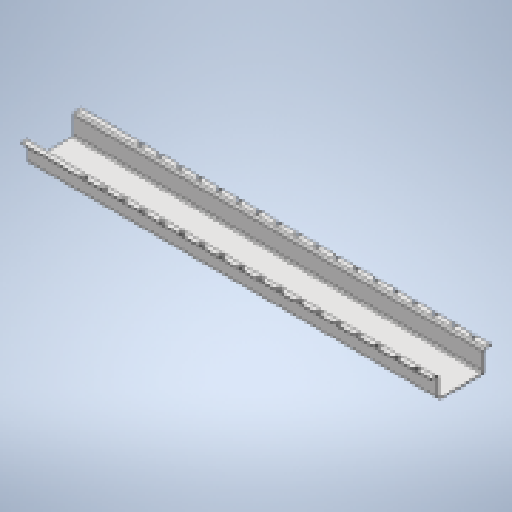
# Autodesk Inventor part: MSC 081 pillar 1_CPY
Saved by Autodesk Inventor 2025 (Build 290162010, 162A)
## iProperties
Created: 2024-06-25
Part Number: MSC 081 pillar 1_CPY
Material: Stainless Steel
Document SubType Name: Sheet Metal
Designer: admin
Density: 8 g/cm^3
Sheet Metal Rule: AISI304 3mm Die 32
Appearance: Default
Author: admin
Autodesk Inventor part; units mm, degrees
ref_plane "YZ Plane" through (0, 0, 0) normal (1, 0, 0) x (0, 1, 0)
ref_plane "XZ Plane" through (0, 0, 0) normal (0, 1, 0) x (-1, 0, 0)
ref_plane "XY Plane" through (0, 0, 0) normal (0, 0, 1) x (1, 0, 0)
sketch3d "3D Sketch1"
sketch "Sketch1" plane through (0, 0, 0) normal (0, 0, 1) x (1, 0, 0)
  line L0 (-675, 75) -> (675, 75)
  line L1 (675, 75) -> (675, -75)
  line L2 (675, -75) -> (-675, -75)
  line L3 (-675, -75) -> (-675, 75)
  line L4 (-675, 75) -> (675, -75) construction
  line L5 (675, 75) -> (-675, -75) construction
  point P0 (0, 0)
  dimension "d5" = 1350
  dimension "d30" = 150
  measures "d5" distance of L1.end L2.end
  measures "d30" distance of L2.end L0.start
extrude "Plate1" add sketch "Sketch1" along normal blind 3
sketch "Sketch6" plane through (675, -72, 0) normal (0, -1, 0) x (1, 0, 0)
  line L0 (-1350, 0) -> (0, 0)
  line L1 (0, 0) -> (0, 70)
  line L2 (0, 70) -> (-1350, 70)
  line L3 (-1350, 70) -> (-1350, 0)
  constraints: 6 end point, 1 horizontal, 1 perpendicular, 1 vertical
edge flange "Flange4" height 70 angle 90 thickness 3 bend radius 5 thickness toward (0, -1, 0) relief round relief width 3 relief depth 1.5 corner gap 5 corner form 0 edges at (0, -75, 3) (0, 75, 3) wall of the first edge with corners at (-675, -72, 0) (675, -72, 0) (675, -72, 70) (-675, -72, 70)
bend "Bend4"
corner "Corner4"
sketch "Sketch9" plane through (-675, -72, 67) normal (0, 0, 1) x (1, 0, 0)
  line L0 (1350, 0) -> (0, 0)
  line L1 (0, 0) -> (0, -25)
  line L2 (0, -25) -> (1350, -25)
  line L3 (1350, -25) -> (1350, 0)
  constraints: 6 end point, 1 horizontal, 1 perpendicular, 1 vertical
edge flange "Flange5" height 22 angle 90 thickness 3 bend radius 5 thickness toward (0, 0, 1) relief round relief width 3 relief depth 1.5 edges at (0, -75, 70) wall of the first edge with corners at (675, -72, 67) (-675, -72, 67) (-675, -97, 67) (675, -97, 67)
bend "Bend5"
corner "Corner5"
sketch "Sketch10" plane through (675, 72, 67) normal (0, 0, 1) x (1, 0, 0)
  line L0 (-1350, 0) -> (0, 0)
  line L1 (0, 0) -> (0, 25)
  line L2 (0, 25) -> (-1350, 25)
  line L3 (-1350, 25) -> (-1350, 0)
  constraints: 6 end point, 1 horizontal, 1 perpendicular, 1 vertical
edge flange "Flange6" height 22 angle 90 thickness 3 bend radius 5 thickness toward (0, 0, 1) relief round relief width 3 relief depth 1.5 edges at (0, 75, 70) wall of the first edge with corners at (-675, 72, 67) (675, 72, 67) (675, 97, 67) (-675, 97, 67)
bend "Bend6"
corner "Corner6"
sketch "Sketch11" plane through (-675, -97, 70) normal (0, 0, 1) x (1, 0, 0)
  circle A0 centre (1304, 8.5) radius 3.5
  line L0 (1350, 17) -> (1350, 0) projected
  point P0 (675, 97)
  point P1 (1350, 8.5)
  point P2 (1350, 8.5)
  dimension "d101" = 46
  dimension "d102" = 7
  constraints: 2 midpoint, 1 centre point, 1 horizontal alignment
  measures "d101" distance of point (1350, 8.5) A0.centre
  measures "d102" diameter of A0
cut "Cut1" [suppressed]
pattern_linear "Rectangular Pattern2" [suppressed]
mirror "Mirror2" [suppressed]
sketch "Sketch12" plane through (0, 0, 3) normal (0, 0, 1) x (1, 0, 0)
  line L0 (675, -97) -> (-675, -97) projected
  line L1 (-675, 97) -> (675, 97) projected
  line L2 (-644.711, -97) -> (-644.711, 97) construction
  arc A0 (-644.711, 97) -> (-644.711, -97) centre (5004.4563, 0) ccw
  line L3 (-675, -97) -> (-675, 97)
  point P0 (0, 0)
  dimension "d117" = 5650
  dimension "d118" = 1319.711
  constraints: 4 end point, 2 point on circle, 2 point on line, 1 centre point, 1 perpendicular, 1 vertical
  measures "d117" radius of A0
  measures "d118" distance of L2.start L0.start
extrude "Extrusion5" cut sketch "Sketch12" along normal through all both and the other way through all
sketch "Sketch13" plane through (-644.9773, -80, 70) normal (0, 0, 1) x (1, 0, 0)
  arc A0 (0, 0) -> (0.2663, -17) centre (5649.4336, 80) ccw projected
  line L0 (1319.9773, -17) -> (0.2663, -17) projected
  line L1 (1319.9773, 0) -> (1319.9773, -17) projected
  line L2 (1319.9773, 0) -> (0, 0) projected
  circle A1 centre (1271.105, -17) radius 5
  circle A2 centre (1273.9773, -9) radius 3.5
  circle A3 centre (1271.105, -17) radius 12
  point P0 (644.9773, 80)
  point P1 (1272.7946, -12.2941)
  point P2 (1275.16, -5.7059)
  point P3 (1283.105, -17)
  point P4 (1276.105, -17)
  point P5 (1259.105, -17)
  point P6 (1266.105, -17)
  dimension "d121" = 10
  dimension "d122" = 46
  dimension "d123" = 8
  dimension "d124" = 7
  constraints: 3 centre point, 2 tangent, 1 coincident, 1 point on line
  measures "d121" diameter of A1
  measures "d122" distance from line of L1 A2.centre
  measures "d123" distance from line of A2.centre L0
  measures "d124" diameter of A2
extrude "Cut2" cut sketch "Sketch13" against normal through all contours A3 A2 A1 L0 | A2 picked at (1267.6356, -9.7193)
pattern_linear "Rectangular Pattern3" count 18 spacing 63 along (-1, 0, 0) of "Cut2"
mirror "Mirror3" about plane through (0, 0, 0) normal (0, 1, 0) of "Cut2", "Rectangular Pattern3"
equation "\"d112\" = Thickness"
equation "\"d127\" = Thickness"
equation "\"d6\" = Thickness"
equation "\"d60\" = BendReliefWidth"
equation "\"d61\" = BendReliefDepth"
equation "\"d62\" = MinimumRemnant"
equation "\"d63\" = TransitionRadius"
equation "\"d66\" = BendRadius"
equation "\"d67\" = CornerReliefSize"
equation "\"d68\" = GapSize"
equation "\"d69\" = JacobiRadiusSize"
equation "\"d81\" = BendReliefWidth"
equation "\"d82\" = BendReliefDepth"
equation "\"d83\" = MinimumRemnant"
equation "\"d84\" = TransitionRadius"
equation "\"d87\" = BendRadius"
equation "\"d88\" = CornerReliefSize"
equation "\"d89\" = GapSize"
equation "\"d90\" = JacobiRadiusSize"
equation "\"d91\" = BendReliefWidth"
equation "\"d92\" = BendReliefDepth"
equation "\"d93\" = MinimumRemnant"
equation "\"d94\" = TransitionRadius"
equation "\"d97\" = BendRadius"
equation "\"d98\" = CornerReliefSize"
equation "\"d99\" = GapSize"
equation "\"d100\" = JacobiRadiusSize"
equation "\"BendReliefWidth\" = Thickness"
equation "\"BendReliefDepth\" = 0.5 * Thickness"
equation "\"CornerReliefSize\" = 4 * Thickness"
equation "\"MinimumRemnant\" = 2 * Thickness"
equation "\"TransitionRadius\" = BendRadius"
equation "\"JacobiRadiusSize\" = BendRadius"
equation "\"GapSize\" = Thickness"
equation "\"Thickness\" = 3"
equation "\"BendRadius\" = 5"
body "Solid1"
